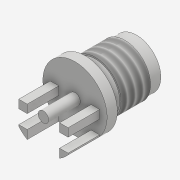
# Autodesk Inventor part: sma-conn
Saved by Autodesk Inventor 2018 (Build 220112000, 112)
## iProperties
Created: 2019-06-30
Part Number: sma-conn
Material: Generic
Document SubType Name: Modeling
Designer: Ocanath
Density: 1 g/cm^3
Appearance: Default
Author: Ocanath
Autodesk Inventor part; units mm, degrees
ref_plane "YZ Plane" through (0, 0, 0) normal (1, 0, 0) x (0, 1, 0)
ref_plane "XZ Plane" through (0, 0, 0) normal (0, 1, 0) x (-1, 0, 0)
sketch "Sketch1" plane through (0, 0, 0) normal (0, 1, 0) x (-1, 0, 0)
  circle A0 centre (0, 0) radius 3
  dimension "d0" = 6
  constraints: 1 centre point, 1 coincident
  measures "d0" diameter of A0
extrude "Extrusion1" add sketch "Sketch1" along normal blind 6.35
sketch "Sketch2" plane through (0, 0, 0) normal (0, -1, 0) x (1, 0, 0)
  circle A0 centre (0, 0) radius 3.965
  dimension "d3" = 7.93
  constraints: 1 centre point, 1 coincident
  measures "d3" diameter of A0
extrude "Extrusion2" add sketch "Sketch2" along normal blind 1.26
sketch "Sketch3" plane through (0, -1.26, 0) normal (0, -1, 0) x (1, 0, 0)
  circle A0 centre (0, 0) radius 0.65
  dimension "d6" = 1.3
  constraints: 1 centre point, 1 coincident
  measures "d6" diameter of A0
extrude "Extrusion3" add sketch "Sketch3" along normal blind 3.9
sketch "Sketch4" plane through (0, -1.26, 0) normal (0, -1, 0) x (1, 0, 0)
  circle A0 centre (0, 0) radius 0.65 projected
  line L0 (0, 0) -> (0, 1.9486) construction
  line L1 (0, 0) -> (1.3232, 0) construction
  line L2 (-3.05, 0.3684) -> (-2, 0.3684)
  line L3 (-2, 0.3684) -> (-2, -0.65)
  line L4 (-2, -0.65) -> (-3.05, -0.65)
  line L5 (-3.05, -0.65) -> (-3.05, 0.3684)
  circle A1 centre (0, 0) radius 2 construction
  line L6 (2, 0.3684) -> (3.05, 0.3684)
  line L7 (3.05, 0.3684) -> (3.05, -0.65)
  line L8 (3.05, -0.65) -> (2, -0.65)
  line L9 (2, -0.65) -> (2, 0.3684)
  dimension "d11" = 4
  dimension "d12" = 6.1
  constraints: 20 end point, 4 parallel, 4 tangent, 3 horizontal, 2 perpendicular, 1 centre point, 1 coincident, 1 collinear, 1 vertical, 1 other
  measures "d11" diameter of A1
  measures "d12" distance between parallel lines of L5 L7
extrude "Extrusion4" add sketch "Sketch4" along normal blind 3.9 contours L2 L3 L4 L5 | L6 L7 L8 L9
sketch "Sketch5" plane through (0, -1.26, 0) normal (0, -1, 0) x (1, 0, 0)
  line L0 (-3.05, -2.35) -> (-2, -2.35)
  line L1 (-2, -2.35) -> (-2, -3.4236)
  line L2 (-3.05, -2.5335) -> (-3.05, -2.35)
  line L3 (-2, 0.3684) -> (-3.05, 0.3684) projected
  line L4 (-3.05, 0.3684) -> (-3.05, -0.65) projected
  line L5 (-3.05, -0.65) -> (-2, -0.65) projected
  line L6 (-2, -0.65) -> (-2, 0.3684) projected
  line L7 (2, -2.35) -> (3.05, -2.35)
  line L8 (3.05, -2.35) -> (3.05, -2.5335)
  line L9 (2, -3.4236) -> (2, -2.35)
  line L10 (2, -0.65) -> (3.05, -0.65) projected
  line L11 (3.05, 0.3684) -> (2, 0.3684) projected
  line L12 (2, 0.3684) -> (2, -0.65) projected
  line L13 (2, -0.65) -> (3.05, -0.65) projected
  line L14 (3.05, -0.65) -> (3.05, 0.3684) projected
  line L15 (2, 0.3684) -> (2, -0.65) projected
  line L16 (-2, -0.65) -> (-2, 0.3684) projected
  circle A0 centre (0, 0) radius 0.65 construction
  line L17 (0, 0) -> (0, 3.0008) construction
  line L18 (3.05, -0.65) -> (3.05, 0.3684) construction
  circle A1 centre (0, 0) radius 3.965 construction
  arc A2 (-3.05, -2.5335) -> (-2, -3.4236) centre (0, 0) ccw
  arc A3 (2, -3.4236) -> (3.05, -2.5335) centre (0, 0) ccw
  dimension "d15" = 1.7
  constraints: 14 end point, 8 point on circle, 4 collinear, 2 centre point, 2 concentric, 2 horizontal, 2 parallel, 2 perpendicular, 1 vertical, 1 other
  measures "d15" distance between parallel lines of L0 L5
extrude "Extrusion5" add sketch "Sketch5" along normal blind 3.9 contours L0 L1 A2 L2 | L7 L8 A3 L9
ref_plane "Work Plane1" through (0, 1.25, 0) normal (0, 1, 0) x (1, 0, 0)
sketch "Sketch6" plane through (0, 1.25, 0) normal (0, 1, 0) x (1, 0, 0)
  circle A0 centre (0, 0) radius 3.175
  dimension "d19" = 6.35
  constraints: 1 centre point, 1 coincident
  measures "d19" diameter of A0
extrude "Extrusion6" add sketch "Sketch6" along normal blind 3.65
thread "Thread1" size "M7x1" class "6g" standard "ANSI Metric M Profile" full length
body "Solid1"
